Autodesk Inventor part; units mm, degrees
(part 2 of 3)
  line L904 (22.3445, 15.4233) -> (22.5183, 15.4736)
  line L905 (22.5183, 15.4736) -> (22.7031, 15.5229)
  line L906 (22.7031, 15.5229) -> (22.8994, 15.5709)
  line L907 (22.8994, 15.5709) -> (23.1087, 15.6175)
  line L908 (23.1087, 15.6175) -> (23.3298, 15.6619)
  line L909 (23.3298, 15.6619) -> (23.5638, 15.7037)
  line L910 (23.5638, 15.7037) -> (23.7624, 15.7353)
  arc A23 (24.1846, 15.0784) -> (23.7624, 15.7353) centre (0, 0) ccw
  line L911 (24.1846, 15.0784) -> (24.0734, 14.9109)
  line L912 (24.0734, 14.9109) -> (23.9381, 14.7154)
  line L913 (23.9381, 14.7154) -> (23.8059, 14.5327)
  line L914 (23.8059, 14.5327) -> (23.6766, 14.3617)
  line L915 (23.6766, 14.3617) -> (23.5513, 14.203)
  line L916 (23.5513, 14.203) -> (23.4297, 14.0554)
  line L917 (23.4297, 14.0554) -> (23.3117, 13.9182)
  line L918 (23.3117, 13.9182) -> (23.1991, 13.7927)
  line L919 (23.1991, 13.7927) -> (23.0918, 13.6779)
  line L920 (23.0918, 13.6779) -> (22.8926, 13.4778)
  line L921 (22.8926, 13.4778) -> (22.6638, 13.2667)
  line L922 (22.6638, 13.2667) -> (22.6103, 13.2101)
  line L923 (22.6103, 13.2101) -> (22.5689, 13.1572)
  line L924 (22.5689, 13.1572) -> (22.5396, 13.1087)
  line L925 (22.5396, 13.1087) -> (22.5221, 13.0649)
  line L926 (22.5221, 13.0649) -> (22.5162, 13.0264)
  line L927 (22.5162, 13.0264) -> (22.5217, 12.9935)
  line L928 (22.5217, 12.9935) -> (22.5383, 12.9627)
  line L929 (22.5383, 12.9627) -> (22.6394, 12.7851)
  line L930 (22.6394, 12.7851) -> (22.7393, 12.6067)
  line L931 (22.7393, 12.6067) -> (22.7571, 12.5766)
  line L932 (22.7571, 12.5766) -> (22.7824, 12.5549)
  line L933 (22.7824, 12.5549) -> (22.8185, 12.5401)
  line L934 (22.8185, 12.5401) -> (22.865, 12.5325)
  line L935 (22.865, 12.5325) -> (22.9217, 12.5325)
  line L936 (22.9217, 12.5325) -> (22.9883, 12.5406)
  line L937 (22.9883, 12.5406) -> (23.0645, 12.5572)
  line L938 (23.0645, 12.5572) -> (23.3634, 12.6442)
  line L939 (23.3634, 12.6442) -> (23.6375, 12.7114)
  line L940 (23.6375, 12.7114) -> (23.7913, 12.7441)
  line L941 (23.7913, 12.7441) -> (23.9569, 12.7757)
  line L942 (23.9569, 12.7757) -> (24.1353, 12.8058)
  line L943 (24.1353, 12.8058) -> (24.3246, 12.8337)
  line L944 (24.3246, 12.8337) -> (24.5251, 12.8591)
  line L945 (24.5251, 12.8591) -> (24.7384, 12.8815)
  line L946 (24.7384, 12.8815) -> (24.9631, 12.9004)
  line L947 (24.9631, 12.9004) -> (25.2003, 12.9153)
  line L948 (25.2003, 12.9153) -> (25.4012, 12.924)
  arc A24 (25.7457, 12.2232) -> (25.4012, 12.924) centre (0, 0) ccw
  line L949 (25.7457, 12.2232) -> (25.6162, 12.0695)
  line L950 (25.6162, 12.0695) -> (25.4595, 11.8907)
  line L951 (25.4595, 11.8907) -> (25.3073, 11.7243)
  line L952 (25.3073, 11.7243) -> (25.1594, 11.5691)
  line L953 (25.1594, 11.5691) -> (25.0168, 11.4258)
  line L954 (25.0168, 11.4258) -> (24.8791, 11.293)
  line L955 (24.8791, 11.293) -> (24.7463, 11.1701)
  line L956 (24.7463, 11.1701) -> (24.6202, 11.0583)
  line L957 (24.6202, 11.0583) -> (24.5004, 10.9564)
  line L958 (24.5004, 10.9564) -> (24.2797, 10.7804)
  line L959 (24.2797, 10.7804) -> (24.0284, 10.5968)
  line L960 (24.0284, 10.5968) -> (23.9687, 10.5466)
  line L961 (23.9687, 10.5466) -> (23.9216, 10.4988)
  line L962 (23.9216, 10.4988) -> (23.8869, 10.4539)
  line L963 (23.8869, 10.4539) -> (23.8646, 10.4124)
  line L964 (23.8646, 10.4124) -> (23.8543, 10.3748)
  line L965 (23.8543, 10.3748) -> (23.856, 10.3416)
  line L966 (23.856, 10.3416) -> (23.869, 10.309)
  line L967 (23.869, 10.309) -> (23.9492, 10.121)
  line L968 (23.9492, 10.121) -> (24.0281, 9.9324)
  line L969 (24.0281, 9.9324) -> (24.0424, 9.9005)
  line L970 (24.0424, 9.9005) -> (24.0651, 9.8761)
  line L971 (24.0651, 9.8761) -> (24.0992, 9.8572)
  line L972 (24.0992, 9.8572) -> (24.1445, 9.8444)
  line L973 (24.1445, 9.8444) -> (24.2009, 9.8379)
  line L974 (24.2009, 9.8379) -> (24.268, 9.8384)
  line L975 (24.268, 9.8384) -> (24.3456, 9.8462)
  line L976 (24.3456, 9.8462) -> (24.6524, 9.8985)
  line L977 (24.6524, 9.8985) -> (24.9324, 9.9341)
  line L978 (24.9324, 9.9341) -> (25.0889, 9.949)
  line L979 (25.0889, 9.949) -> (25.2571, 9.9615)
  line L980 (25.2571, 9.9615) -> (25.4378, 9.9711)
  line L981 (25.4378, 9.9711) -> (25.6289, 9.9773)
  line L982 (25.6289, 9.9773) -> (25.8311, 9.9796)
  line L983 (25.8311, 9.9796) -> (26.0455, 9.9776)
  line L984 (26.0455, 9.9776) -> (26.2709, 9.9707)
  line L985 (26.2709, 9.9707) -> (26.5083, 9.9585)
  line L986 (26.5083, 9.9585) -> (26.7088, 9.9443)
  arc A25 (26.9713, 9.2088) -> (26.7088, 9.9443) centre (0, 0) ccw
  line L987 (26.9713, 9.2088) -> (26.825, 9.0708)
  line L988 (26.825, 9.0708) -> (26.649, 8.9111)
  line L989 (26.649, 8.9111) -> (26.4788, 8.7631)
  line L990 (26.4788, 8.7631) -> (26.3141, 8.6258)
  line L991 (26.3141, 8.6258) -> (26.1562, 8.4996)
  line L992 (26.1562, 8.4996) -> (26.0043, 8.3834)
  line L993 (26.0043, 8.3834) -> (25.8583, 8.2765)
  line L994 (25.8583, 8.2765) -> (25.7202, 8.1797)
  line L995 (25.7202, 8.1797) -> (25.5896, 8.0922)
  line L996 (25.5896, 8.0922) -> (25.3504, 7.9424)
  line L997 (25.3504, 7.9424) -> (25.0797, 7.7887)
  line L998 (25.0797, 7.7887) -> (25.0147, 7.7456)
  line L999 (25.0147, 7.7456) -> (24.9625, 7.7035)
  line L1000 (24.9625, 7.7035) -> (24.9229, 7.6629)
  line L1001 (24.9229, 7.6629) -> (24.8959, 7.6242)
  line L1002 (24.8959, 7.6242) -> (24.8815, 7.588)
  line L1003 (24.8815, 7.588) -> (24.8794, 7.5548)
  line L1004 (24.8794, 7.5548) -> (24.8885, 7.521)
  line L1005 (24.8885, 7.521) -> (24.9468, 7.325)
  line L1006 (24.9468, 7.325) -> (25.0037, 7.1287)
  line L1007 (25.0037, 7.1287) -> (25.0143, 7.0953)
  line L1008 (25.0143, 7.0953) -> (25.034, 7.0685)
  line L1009 (25.034, 7.0685) -> (25.0657, 7.0459)
  line L1010 (25.0657, 7.0459) -> (25.1093, 7.0279)
  line L1011 (25.1093, 7.0279) -> (25.1646, 7.0151)
  line L1012 (25.1646, 7.0151) -> (25.2313, 7.0079)
  line L1013 (25.2313, 7.0079) -> (25.3092, 7.0069)
  line L1014 (25.3092, 7.0069) -> (25.6201, 7.0238)
  line L1015 (25.6201, 7.0238) -> (25.9023, 7.0272)
  line L1016 (25.9023, 7.0272) -> (26.0595, 7.0242)
  line L1017 (26.0595, 7.0242) -> (26.228, 7.0175)
  line L1018 (26.228, 7.0175) -> (26.4086, 7.0064)
  line L1019 (26.4086, 7.0064) -> (26.5992, 6.9908)
  line L1020 (26.5992, 6.9908) -> (26.8003, 6.97)
  line L1021 (26.8003, 6.97) -> (27.0131, 6.9436)
  line L1022 (27.0131, 6.9436) -> (27.2362, 6.9111)
  line L1023 (27.2362, 6.9111) -> (27.4707, 6.8718)
  line L1024 (27.4707, 6.8718) -> (27.6683, 6.8349)
  arc A26 (27.8452, 6.0743) -> (27.6683, 6.8349) centre (0, 0) ccw
  line L1025 (27.8452, 6.0743) -> (27.6842, 5.9539)
  line L1026 (27.6842, 5.9539) -> (27.4911, 5.8152)
  line L1027 (27.4911, 5.8152) -> (27.3052, 5.6876)
  line L1028 (27.3052, 5.6876) -> (27.1259, 5.57)
  line L1029 (27.1259, 5.57) -> (26.9546, 5.4626)
  line L1030 (26.9546, 5.4626) -> (26.7904, 5.3644)
  line L1031 (26.7904, 5.3644) -> (26.6332, 5.2749)
  line L1032 (26.6332, 5.2749) -> (26.485, 5.1945)
  line L1033 (26.485, 5.1945) -> (26.3453, 5.1224)
  line L1034 (26.3453, 5.1224) -> (26.0905, 5.0009)
  line L1035 (26.0905, 5.0009) -> (25.8041, 4.879)
  line L1036 (25.8041, 4.879) -> (25.7346, 4.8437)
  line L1037 (25.7346, 4.8437) -> (25.6779, 4.8078)
  line L1038 (25.6779, 4.8078) -> (25.6339, 4.7719)
  line L1039 (25.6339, 4.7719) -> (25.6028, 4.7366)
  line L1040 (25.6028, 4.7366) -> (25.5842, 4.7023)
  line L1041 (25.5842, 4.7023) -> (25.5784, 4.6695)
  line L1042 (25.5784, 4.6695) -> (25.5836, 4.6349)
  line L1043 (25.5836, 4.6349) -> (25.6192, 4.4336)
  line L1044 (25.6192, 4.4336) -> (25.6534, 4.232)
  line L1045 (25.6534, 4.232) -> (25.66, 4.1976)
  line L1046 (25.66, 4.1976) -> (25.6766, 4.1688)
  line L1047 (25.6766, 4.1688) -> (25.7055, 4.1427)
  line L1048 (25.7055, 4.1427) -> (25.7468, 4.1199)
  line L1049 (25.7468, 4.1199) -> (25.8002, 4.1008)
  line L1050 (25.8002, 4.1008) -> (25.8657, 4.0861)
  line L1051 (25.8657, 4.0861) -> (25.943, 4.0762)
  line L1052 (25.943, 4.0762) -> (26.2537, 4.0576)
  line L1053 (26.2537, 4.0576) -> (26.5345, 4.0288)
  line L1054 (26.5345, 4.0288) -> (26.6903, 4.0079)
  line L1055 (26.6903, 4.0079) -> (26.857, 3.982)
  line L1056 (26.857, 3.982) -> (27.0351, 3.9504)
  line L1057 (27.0351, 3.9504) -> (27.2227, 3.9131)
  line L1058 (27.2227, 3.9131) -> (27.4201, 3.8696)
  line L1059 (27.4201, 3.8696) -> (27.6285, 3.8191)
  line L1060 (27.6285, 3.8191) -> (27.8465, 3.7613)
  line L1061 (27.8465, 3.7613) -> (28.075, 3.6956)
  line L1062 (28.075, 3.6956) -> (28.2671, 3.6364)
  arc A27 (28.3561, 2.8605) -> (28.2671, 3.6364) centre (0, 0) ccw
  line L1063 (28.3561, 2.8605) -> (28.1824, 2.7593)
  line L1064 (28.1824, 2.7593) -> (27.9748, 2.6436)
  line L1065 (27.9748, 2.6436) -> (27.7755, 2.538)
  line L1066 (27.7755, 2.538) -> (27.584, 2.4415)
  line L1067 (27.584, 2.4415) -> (27.4016, 2.3544)
  line L1068 (27.4016, 2.3544) -> (27.2273, 2.2756)
  line L1069 (27.2273, 2.2756) -> (27.0609, 2.2045)
  line L1070 (27.0609, 2.2045) -> (26.9045, 2.1416)
  line L1071 (26.9045, 2.1416) -> (26.7575, 2.0859)
  line L1072 (26.7575, 2.0859) -> (26.4905, 1.9943)
  line L1073 (26.4905, 1.9943) -> (26.192, 1.9058)
  line L1074 (26.192, 1.9058) -> (26.119, 1.8786)
  line L1075 (26.119, 1.8786) -> (26.0586, 1.8494)
  line L1076 (26.0586, 1.8494) -> (26.0108, 1.8188)
  line L1077 (26.0108, 1.8188) -> (25.9758, 1.7872)
  line L1078 (25.9758, 1.7872) -> (25.9535, 1.7552)
  line L1079 (25.9535, 1.7552) -> (25.9439, 1.7234)
  line L1080 (25.9439, 1.7234) -> (25.9452, 1.6884)
  line L1081 (25.9452, 1.6884) -> (25.9576, 1.4843)
  line L1082 (25.9576, 1.4843) -> (25.9685, 1.2802)
  line L1083 (25.9685, 1.2802) -> (25.9713, 1.2453)
  line L1084 (25.9713, 1.2453) -> (25.9844, 1.2147)
  line L1085 (25.9844, 1.2147) -> (26.0102, 1.1855)
  line L1086 (26.0102, 1.1855) -> (26.0486, 1.1581)
  line L1087 (26.0486, 1.1581) -> (26.0995, 1.1331)
  line L1088 (26.0995, 1.1331) -> (26.1629, 1.111)
  line L1089 (26.1629, 1.111) -> (26.2385, 1.0923)
  line L1090 (26.2385, 1.0923) -> (26.5451, 1.0384)
  line L1091 (26.5451, 1.0384) -> (26.8208, 0.9778)
  line L1092 (26.8208, 0.9778) -> (26.9732, 0.9393)
  line L1093 (26.9732, 0.9393) -> (27.1358, 0.8945)
  line L1094 (27.1358, 0.8945) -> (27.3092, 0.8429)
  line L1095 (27.3092, 0.8429) -> (27.4913, 0.7845)
  line L1096 (27.4913, 0.7845) -> (27.6825, 0.7187)
  line L1097 (27.6825, 0.7187) -> (27.8838, 0.6447)
  line L1098 (27.8838, 0.6447) -> (28.0938, 0.5625)
  line L1099 (28.0938, 0.5625) -> (28.3132, 0.4712)
  line L1100 (28.3132, 0.4712) -> (28.4973, 0.3904)
  arc A28 (28.4973, -0.3904) -> (28.4973, 0.3904) centre (0, 0) ccw
  line L1101 (28.4973, -0.3904) -> (28.3132, -0.4712)
  line L1102 (28.3132, -0.4712) -> (28.0938, -0.5625)
  line L1103 (28.0938, -0.5625) -> (27.8838, -0.6447)
  line L1104 (27.8838, -0.6447) -> (27.6825, -0.7187)
  line L1105 (27.6825, -0.7187) -> (27.4913, -0.7845)
  line L1106 (27.4913, -0.7845) -> (27.3092, -0.8429)
  line L1107 (27.3092, -0.8429) -> (27.1358, -0.8945)
  line L1108 (27.1358, -0.8945) -> (26.9732, -0.9393)
  line L1109 (26.9732, -0.9393) -> (26.8208, -0.9778)
  line L1110 (26.8208, -0.9778) -> (26.5451, -1.0384)
  line L1111 (26.5451, -1.0384) -> (26.2385, -1.0923)
  line L1112 (26.2385, -1.0923) -> (26.1629, -1.111)
  line L1113 (26.1629, -1.111) -> (26.0995, -1.1331)
  line L1114 (26.0995, -1.1331) -> (26.0486, -1.1581)
  line L1115 (26.0486, -1.1581) -> (26.0102, -1.1855)
  line L1116 (26.0102, -1.1855) -> (25.9844, -1.2147)
  line L1117 (25.9844, -1.2147) -> (25.9713, -1.2453)
  line L1118 (25.9713, -1.2453) -> (25.9685, -1.2802)
  line L1119 (25.9685, -1.2802) -> (25.9576, -1.4843)
  line L1120 (25.9576, -1.4843) -> (25.9452, -1.6884)
  line L1121 (25.9452, -1.6884) -> (25.9439, -1.7234)
  line L1122 (25.9439, -1.7234) -> (25.9535, -1.7552)
  line L1123 (25.9535, -1.7552) -> (25.9758, -1.7872)
  line L1124 (25.9758, -1.7872) -> (26.0108, -1.8188)
  line L1125 (26.0108, -1.8188) -> (26.0586, -1.8494)
  line L1126 (26.0586, -1.8494) -> (26.119, -1.8786)
  line L1127 (26.119, -1.8786) -> (26.192, -1.9058)
  line L1128 (26.192, -1.9058) -> (26.4905, -1.9943)
  line L1129 (26.4905, -1.9943) -> (26.7575, -2.0859)
  line L1130 (26.7575, -2.0859) -> (26.9045, -2.1416)
  line L1131 (26.9045, -2.1416) -> (27.0609, -2.2045)
  line L1132 (27.0609, -2.2045) -> (27.2273, -2.2756)
  line L1133 (27.2273, -2.2756) -> (27.4016, -2.3544)
  line L1134 (27.4016, -2.3544) -> (27.584, -2.4415)
  line L1135 (27.584, -2.4415) -> (27.7755, -2.538)
  line L1136 (27.7755, -2.538) -> (27.9748, -2.6436)
  line L1137 (27.9748, -2.6436) -> (28.1824, -2.7593)
  line L1138 (28.1824, -2.7593) -> (28.3561, -2.8605)
  arc A29 (28.2671, -3.6364) -> (28.3561, -2.8605) centre (0, 0) ccw
  line L1139 (28.2671, -3.6364) -> (28.075, -3.6956)
  line L1140 (28.075, -3.6956) -> (27.8465, -3.7613)
  line L1141 (27.8465, -3.7613) -> (27.6285, -3.8191)
  line L1142 (27.6285, -3.8191) -> (27.4201, -3.8696)
  line L1143 (27.4201, -3.8696) -> (27.2227, -3.9131)
  line L1144 (27.2227, -3.9131) -> (27.0351, -3.9504)
  line L1145 (27.0351, -3.9504) -> (26.857, -3.982)
  line L1146 (26.857, -3.982) -> (26.6903, -4.0079)
  line L1147 (26.6903, -4.0079) -> (26.5345, -4.0288)
  line L1148 (26.5345, -4.0288) -> (26.2537, -4.0576)
  line L1149 (26.2537, -4.0576) -> (25.943, -4.0762)
  line L1150 (25.943, -4.0762) -> (25.8657, -4.0861)
  line L1151 (25.8657, -4.0861) -> (25.8002, -4.1008)
  line L1152 (25.8002, -4.1008) -> (25.7468, -4.1199)
  line L1153 (25.7468, -4.1199) -> (25.7055, -4.1427)
  line L1154 (25.7055, -4.1427) -> (25.6766, -4.1688)
  line L1155 (25.6766, -4.1688) -> (25.66, -4.1976)
  line L1156 (25.66, -4.1976) -> (25.6534, -4.232)
  line L1157 (25.6534, -4.232) -> (25.6192, -4.4336)
  line L1158 (25.6192, -4.4336) -> (25.5836, -4.6349)
  line L1159 (25.5836, -4.6349) -> (25.5784, -4.6695)
  line L1160 (25.5784, -4.6695) -> (25.5842, -4.7023)
  line L1161 (25.5842, -4.7023) -> (25.6028, -4.7366)
  line L1162 (25.6028, -4.7366) -> (25.6339, -4.7719)
  line L1163 (25.6339, -4.7719) -> (25.6779, -4.8078)
  line L1164 (25.6779, -4.8078) -> (25.7346, -4.8437)
  line L1165 (25.7346, -4.8437) -> (25.8041, -4.879)
  line L1166 (25.8041, -4.879) -> (26.0905, -5.0009)
  line L1167 (26.0905, -5.0009) -> (26.3453, -5.1224)
  line L1168 (26.3453, -5.1224) -> (26.485, -5.1945)
  line L1169 (26.485, -5.1945) -> (26.6332, -5.2749)
  line L1170 (26.6332, -5.2749) -> (26.7904, -5.3644)
  line L1171 (26.7904, -5.3644) -> (26.9546, -5.4626)
  line L1172 (26.9546, -5.4626) -> (27.1259, -5.57)
  line L1173 (27.1259, -5.57) -> (27.3052, -5.6876)
  line L1174 (27.3052, -5.6876) -> (27.4911, -5.8152)
  line L1175 (27.4911, -5.8152) -> (27.6842, -5.9539)
  line L1176 (27.6842, -5.9539) -> (27.8452, -6.0742)
  arc A30 (27.6683, -6.8349) -> (27.8452, -6.0742) centre (0, 0) ccw
  line L1177 (27.6683, -6.8349) -> (27.4707, -6.8718)
  line L1178 (27.4707, -6.8718) -> (27.2362, -6.9111)
  line L1179 (27.2362, -6.9111) -> (27.0131, -6.9436)
  line L1180 (27.0131, -6.9436) -> (26.8003, -6.97)
  line L1181 (26.8003, -6.97) -> (26.5992, -6.9908)
  line L1182 (26.5992, -6.9908) -> (26.4086, -7.0064)
  line L1183 (26.4086, -7.0064) -> (26.228, -7.0175)
  line L1184 (26.228, -7.0175) -> (26.0595, -7.0242)
  line L1185 (26.0595, -7.0242) -> (25.9023, -7.0272)
  line L1186 (25.9023, -7.0272) -> (25.6201, -7.0238)
  line L1187 (25.6201, -7.0238) -> (25.3092, -7.0069)
  line L1188 (25.3092, -7.0069) -> (25.2313, -7.0079)
  line L1189 (25.2313, -7.0079) -> (25.1646, -7.0151)
  line L1190 (25.1646, -7.0151) -> (25.1093, -7.0279)
  line L1191 (25.1093, -7.0279) -> (25.0657, -7.0459)
  line L1192 (25.0657, -7.0459) -> (25.034, -7.0685)
  line L1193 (25.034, -7.0685) -> (25.0143, -7.0953)
  line L1194 (25.0143, -7.0953) -> (25.0037, -7.1287)
  line L1195 (25.0037, -7.1287) -> (24.9468, -7.325)
  line L1196 (24.9468, -7.325) -> (24.8885, -7.521)
  line L1197 (24.8885, -7.521) -> (24.8794, -7.5548)
  line L1198 (24.8794, -7.5548) -> (24.8815, -7.588)
  line L1199 (24.8815, -7.588) -> (24.8959, -7.6242)
  line L1200 (24.8959, -7.6242) -> (24.9229, -7.6629)
  line L1201 (24.9229, -7.6629) -> (24.9625, -7.7035)
  line L1202 (24.9625, -7.7035) -> (25.0147, -7.7456)
  line L1203 (25.0147, -7.7456) -> (25.0797, -7.7887)
  line L1204 (25.0797, -7.7887) -> (25.3504, -7.9424)
  line L1205 (25.3504, -7.9424) -> (25.5896, -8.0922)
  line L1206 (25.5896, -8.0922) -> (25.7202, -8.1797)
  line L1207 (25.7202, -8.1797) -> (25.8583, -8.2765)
  line L1208 (25.8583, -8.2765) -> (26.0043, -8.3834)
  line L1209 (26.0043, -8.3834) -> (26.1562, -8.4996)
  line L1210 (26.1562, -8.4996) -> (26.3141, -8.6258)
  line L1211 (26.3141, -8.6258) -> (26.4788, -8.7631)
  line L1212 (26.4788, -8.7631) -> (26.649, -8.9111)
  line L1213 (26.649, -8.9111) -> (26.825, -9.0708)
  line L1214 (26.825, -9.0708) -> (26.9713, -9.2088)
  arc A31 (26.7088, -9.9443) -> (26.9713, -9.2088) centre (0, 0) ccw
  line L1215 (26.7088, -9.9443) -> (26.5083, -9.9585)
  line L1216 (26.5083, -9.9585) -> (26.2709, -9.9707)
  line L1217 (26.2709, -9.9707) -> (26.0455, -9.9776)
  line L1218 (26.0455, -9.9776) -> (25.8311, -9.9796)
  line L1219 (25.8311, -9.9796) -> (25.6289, -9.9773)
  line L1220 (25.6289, -9.9773) -> (25.4378, -9.9711)
  line L1221 (25.4378, -9.9711) -> (25.2571, -9.9615)
  line L1222 (25.2571, -9.9615) -> (25.0889, -9.949)
  line L1223 (25.0889, -9.949) -> (24.9324, -9.9341)
  line L1224 (24.9324, -9.9341) -> (24.6524, -9.8985)
  line L1225 (24.6524, -9.8985) -> (24.3456, -9.8462)
  line L1226 (24.3456, -9.8462) -> (24.268, -9.8384)
  line L1227 (24.268, -9.8384) -> (24.2009, -9.8379)
  line L1228 (24.2009, -9.8379) -> (24.1445, -9.8444)
  line L1229 (24.1445, -9.8444) -> (24.0992, -9.8572)
  line L1230 (24.0992, -9.8572) -> (24.0651, -9.8761)
  line L1231 (24.0651, -9.8761) -> (24.0424, -9.9005)
  line L1232 (24.0424, -9.9005) -> (24.0281, -9.9324)
  line L1233 (24.0281, -9.9324) -> (23.9492, -10.121)
  line L1234 (23.9492, -10.121) -> (23.869, -10.309)
  line L1235 (23.869, -10.309) -> (23.856, -10.3416)
  line L1236 (23.856, -10.3416) -> (23.8543, -10.3748)
  line L1237 (23.8543, -10.3748) -> (23.8646, -10.4124)
  line L1238 (23.8646, -10.4124) -> (23.8869, -10.4539)
  line L1239 (23.8869, -10.4539) -> (23.9216, -10.4988)
  line L1240 (23.9216, -10.4988) -> (23.9687, -10.5466)
  line L1241 (23.9687, -10.5466) -> (24.0284, -10.5968)
  line L1242 (24.0284, -10.5968) -> (24.2797, -10.7804)
  line L1243 (24.2797, -10.7804) -> (24.5004, -10.9564)
  line L1244 (24.5004, -10.9564) -> (24.6202, -11.0583)
  line L1245 (24.6202, -11.0583) -> (24.7463, -11.1701)
  line L1246 (24.7463, -11.1701) -> (24.8791, -11.293)
  line L1247 (24.8791, -11.293) -> (25.0168, -11.4258)
  line L1248 (25.0168, -11.4258) -> (25.1594, -11.5691)
  line L1249 (25.1594, -11.5691) -> (25.3073, -11.7243)
  line L1250 (25.3073, -11.7243) -> (25.4595, -11.8907)
  line L1251 (25.4595, -11.8907) -> (25.6162, -12.0695)
  line L1252 (25.6162, -12.0695) -> (25.7457, -12.2232)
  arc A32 (25.4012, -12.924) -> (25.7457, -12.2232) centre (0, 0) ccw
  line L1253 (25.4012, -12.924) -> (25.2003, -12.9153)
  line L1254 (25.2003, -12.9153) -> (24.9631, -12.9004)
  line L1255 (24.9631, -12.9004) -> (24.7384, -12.8815)
  line L1256 (24.7384, -12.8815) -> (24.5251, -12.8591)
  line L1257 (24.5251, -12.8591) -> (24.3246, -12.8337)
  line L1258 (24.3246, -12.8337) -> (24.1353, -12.8058)
  line L1259 (24.1353, -12.8058) -> (23.9569, -12.7757)
  line L1260 (23.9569, -12.7757) -> (23.7913, -12.7441)
  line L1261 (23.7913, -12.7441) -> (23.6375, -12.7114)
  line L1262 (23.6375, -12.7114) -> (23.3634, -12.6442)
  line L1263 (23.3634, -12.6442) -> (23.0645, -12.5572)
  line L1264 (23.0645, -12.5572) -> (22.9883, -12.5406)
  line L1265 (22.9883, -12.5406) -> (22.9217, -12.5325)
  line L1266 (22.9217, -12.5325) -> (22.865, -12.5325)
  line L1267 (22.865, -12.5325) -> (22.8185, -12.5401)
  line L1268 (22.8185, -12.5401) -> (22.7824, -12.5549)
  line L1269 (22.7824, -12.5549) -> (22.7571, -12.5766)
  line L1270 (22.7571, -12.5766) -> (22.7393, -12.6067)
  line L1271 (22.7393, -12.6067) -> (22.6394, -12.7851)
  line L1272 (22.6394, -12.7851) -> (22.5383, -12.9627)
  line L1273 (22.5383, -12.9627) -> (22.5217, -12.9935)
  line L1274 (22.5217, -12.9935) -> (22.5162, -13.0264)
  line L1275 (22.5162, -13.0264) -> (22.5221, -13.0649)
  line L1276 (22.5221, -13.0649) -> (22.5396, -13.1087)
  line L1277 (22.5396, -13.1087) -> (22.5689, -13.1572)
  line L1278 (22.5689, -13.1572) -> (22.6103, -13.2101)
  line L1279 (22.6103, -13.2101) -> (22.6638, -13.2667)
  line L1280 (22.6638, -13.2667) -> (22.8926, -13.4778)
  line L1281 (22.8926, -13.4778) -> (23.0918, -13.6779)
  line L1282 (23.0918, -13.6779) -> (23.1991, -13.7927)
  line L1283 (23.1991, -13.7927) -> (23.3117, -13.9182)
  line L1284 (23.3117, -13.9182) -> (23.4297, -14.0554)
  line L1285 (23.4297, -14.0554) -> (23.5513, -14.203)
  line L1286 (23.5513, -14.203) -> (23.6766, -14.3617)
  line L1287 (23.6766, -14.3617) -> (23.8059, -14.5327)
  line L1288 (23.8059, -14.5327) -> (23.9381, -14.7154)
  line L1289 (23.9381, -14.7154) -> (24.0734, -14.9109)
  line L1290 (24.0734, -14.9109) -> (24.1846, -15.0784)
  arc A33 (23.7624, -15.7353) -> (24.1846, -15.0784) centre (0, 0) ccw
  line L1291 (23.7624, -15.7353) -> (23.5638, -15.7037)
  line L1292 (23.5638, -15.7037) -> (23.3298, -15.6619)
  line L1293 (23.3298, -15.6619) -> (23.1087, -15.6175)
  line L1294 (23.1087, -15.6175) -> (22.8994, -15.5709)
  line L1295 (22.8994, -15.5709) -> (22.7031, -15.5229)
  line L1296 (22.7031, -15.5229) -> (22.5183, -15.4736)
  line L1297 (22.5183, -15.4736) -> (22.3445, -15.4233)
  line L1298 (22.3445, -15.4233) -> (22.1835, -15.373)
  line L1299 (22.1835, -15.373) -> (22.0345, -15.323)
  line L1300 (22.0345, -15.323) -> (21.7698, -15.225)
  line L1301 (21.7698, -15.225) -> (21.4827, -15.1045)
  line L1302 (21.4827, -15.1045) -> (21.4089, -15.0794)
  line L1303 (21.4089, -15.0794) -> (21.3437, -15.0637)
  line L1304 (21.3437, -15.0637) -> (21.2874, -15.0572)
  line L1305 (21.2874, -15.0572) -> (21.2403, -15.0594)
  line L1306 (21.2403, -15.0594) -> (21.2028, -15.0701)
  line L1307 (21.2028, -15.0701) -> (21.1752, -15.0887)
  line L1308 (21.1752, -15.0887) -> (21.154, -15.1166)
  line L1309 (21.154, -15.1166) -> (21.0344, -15.2824)
  line L1310 (21.0344, -15.2824) -> (20.9137, -15.4474)
  line L1311 (20.9137, -15.4474) -> (20.8937, -15.4761)
  line L1312 (20.8937, -15.4761) -> (20.8845, -15.5081)
  line L1313 (20.8845, -15.5081) -> (20.886, -15.5471)
  line L1314 (20.886, -15.5471) -> (20.8984, -15.5926)
  line L1315 (20.8984, -15.5926) -> (20.922, -15.6441)
  line L1316 (20.922, -15.6441) -> (20.957, -15.7013)
  line L1317 (20.957, -15.7013) -> (21.0038, -15.7637)
  line L1318 (21.0038, -15.7637) -> (21.207, -15.9995)
  line L1319 (21.207, -15.9995) -> (21.3821, -16.221)
  line L1320 (21.3821, -16.221) -> (21.4757, -16.3473)
  line L1321 (21.4757, -16.3473) -> (21.5732, -16.4848)
  line L1322 (21.5732, -16.4848) -> (21.6748, -16.6345)
  line L1323 (21.6748, -16.6345) -> (21.7788, -16.7951)
  line L1324 (21.7788, -16.7951) -> (21.8851, -16.967)
  line L1325 (21.8851, -16.967) -> (21.9941, -17.1517)
  line L1326 (21.9941, -17.1517) -> (22.1046, -17.3482)
  line L1327 (22.1046, -17.3482) -> (22.2167, -17.5578)
  line L1328 (22.2167, -17.5578) -> (22.3081, -17.7369)
  arc A34 (21.8138, -18.3414) -> (22.3081, -17.7369) centre (0, 0) ccw
  line L1329 (21.8138, -18.3414) -> (21.6202, -18.2874)
  line L1330 (21.6202, -18.2874) -> (21.3925, -18.2192)
  line L1331 (21.3925, -18.2192) -> (21.1779, -18.1499)
  line L1332 (21.1779, -18.1499) -> (20.9752, -18.0798)
  line L1333 (20.9752, -18.0798) -> (20.7856, -18.0097)
  line L1334 (20.7856, -18.0097) -> (20.6076, -17.9396)
  line L1335 (20.6076, -17.9396) -> (20.4407, -17.8698)
  line L1336 (20.4407, -17.8698) -> (20.2865, -17.8015)
  line L1337 (20.2865, -17.8015) -> (20.1442, -17.7349)
  line L1338 (20.1442, -17.7349) -> (19.8924, -17.6073)
  line L1339 (19.8924, -17.6073) -> (19.6209, -17.4549)
  line L1340 (19.6209, -17.4549) -> (19.5505, -17.4215)
  line L1341 (19.5505, -17.4215) -> (19.4874, -17.3985)
  line L1342 (19.4874, -17.3985) -> (19.4322, -17.3856)
  line L1343 (19.4322, -17.3856) -> (19.3852, -17.3825)
  line L1344 (19.3852, -17.3825) -> (19.3467, -17.3888)
  line L1345 (19.3467, -17.3888) -> (19.3172, -17.4041)
  line L1346 (19.3172, -17.4041) -> (19.293, -17.4295)
  line L1347 (19.293, -17.4295) -> (19.1553, -17.5805)
  line L1348 (19.1553, -17.5805) -> (19.0165, -17.7307)
  line L1349 (19.0165, -17.7307) -> (18.9934, -17.757)
  line L1350 (18.9934, -17.757) -> (18.9806, -17.7877)
  line L1351 (18.9806, -17.7877) -> (18.9776, -17.8266)
  line L1352 (18.9776, -17.8266) -> (18.9847, -17.8732)
  line L1353 (18.9847, -17.8732) -> (19.0023, -17.9271)
  line L1354 (19.0023, -17.9271) -> (19.0306, -17.9879)
  line L1355 (19.0306, -17.9879) -> (19.07, -18.0552)
  line L1356 (19.07, -18.0552) -> (19.245, -18.3126)
  line L1357 (19.245, -18.3126) -> (19.3937, -18.5526)
  line L1358 (19.3937, -18.5526) -> (19.4722, -18.6887)
  line L1359 (19.4722, -18.6887) -> (19.5535, -18.8365)
  line L1360 (19.5535, -18.8365) -> (19.6373, -18.9968)
  line L1361 (19.6373, -18.9968) -> (19.7223, -19.1682)
  line L1362 (19.7223, -19.1682) -> (19.8084, -19.3511)
  line L1363 (19.8084, -19.3511) -> (19.8956, -19.547)
  line L1364 (19.8956, -19.547) -> (19.983, -19.7549)
  line L1365 (19.983, -19.7549) -> (20.0705, -19.9759)
  line L1366 (20.0705, -19.9759) -> (20.1409, -20.1642)
  arc A35 (19.5809, -20.7085) -> (20.1409, -20.1642) centre (0, 0) ccw
  line L1367 (19.5809, -20.7085) -> (19.3946, -20.6327)
  line L1368 (19.3946, -20.6327) -> (19.1762, -20.539)
  line L1369 (19.1762, -20.539) -> (18.9709, -20.4457)
  line L1370 (18.9709, -20.4457) -> (18.7776, -20.3529)
  line L1371 (18.7776, -20.3529) -> (18.5972, -20.2616)
  line L1372 (18.5972, -20.2616) -> (18.4283, -20.1717)
  line L1373 (18.4283, -20.1717) -> (18.2705, -20.0834)
  line L1374 (18.2705, -20.0834) -> (18.1251, -19.998)
  line L1375 (18.1251, -19.998) -> (17.9912, -19.9155)
  line L1376 (17.9912, -19.9155) -> (17.7556, -19.7601)
  line L1377 (17.7556, -19.7601) -> (17.5033, -19.5778)
  line L1378 (17.5033, -19.5778) -> (17.4371, -19.5365)
  line L1379 (17.4371, -19.5365) -> (17.3771, -19.5065)
  line L1380 (17.3771, -19.5065) -> (17.3237, -19.4874)
  line L1381 (17.3237, -19.4874) -> (17.2774, -19.4789)
  line L1382 (17.2774, -19.4789) -> (17.2384, -19.4808)
  line L1383 (17.2384, -19.4808) -> (17.2073, -19.4927)
  line L1384 (17.2073, -19.4927) -> (17.1804, -19.5151)
  line L1385 (17.1804, -19.5151) -> (17.0264, -19.6495)
  line L1386 (17.0264, -19.6495) -> (16.8714, -19.7828)
  line L1387 (16.8714, -19.7828) -> (16.8454, -19.8063)
  line L1388 (16.8454, -19.8063) -> (16.8292, -19.8354)
  line L1389 (16.8292, -19.8354) -> (16.8218, -19.8736)
  line L1390 (16.8218, -19.8736) -> (16.8236, -19.9208)
  line L1391 (16.8236, -19.9208) -> (16.8349, -19.9763)
  line L1392 (16.8349, -19.9763) -> (16.8561, -20.04)
  line L1393 (16.8561, -20.04) -> (16.8875, -20.1113)
  line L1394 (16.8875, -20.1113) -> (17.0321, -20.387)
  line L1395 (17.0321, -20.387) -> (17.1524, -20.6424)
  line L1396 (17.1524, -20.6424) -> (17.215, -20.7866)
  line L1397 (17.215, -20.7866) -> (17.2788, -20.9427)
  line L1398 (17.2788, -20.9427) -> (17.3438, -21.1115)
  line L1399 (17.3438, -21.1115) -> (17.4088, -21.2914)
  line L1400 (17.4088, -21.2914) -> (17.4734, -21.483)
  line L1401 (17.4734, -21.483) -> (17.5377, -21.6875)
  line L1402 (17.5377, -21.6875) -> (17.6009, -21.904)
  line L1403 (17.6009, -21.904) -> (17.6626, -22.1336)
  line L1404 (17.6626, -22.1336) -> (17.711, -22.3287)
  arc A36 (17.0926, -22.8055) -> (17.711, -22.3287) centre (0, 0) ccw
  line L1405 (17.0926, -22.8055) -> (16.9163, -22.7091)
  line L1406 (16.9163, -22.7091) -> (16.7099, -22.591)
  line L1407 (16.7099, -22.591) -> (16.5166, -22.4749)
  line L1408 (16.5166, -22.4749) -> (16.3351, -22.3607)
  line L1409 (16.3351, -22.3607) -> (16.1663, -22.2495)
  line L1410 (16.1663, -22.2495) -> (16.0088, -22.1409)
  line L1411 (16.0088, -22.1409) -> (15.862, -22.0352)
  line L1412 (15.862, -22.0352) -> (15.7273, -21.9337)
  line L1413 (15.7273, -21.9337) -> (15.6038, -21.8366)
  line L1414 (15.6038, -21.8366) -> (15.3874, -21.6553)
  line L1415 (15.3874, -21.6553) -> (15.1575, -21.4454)
  line L1416 (15.1575, -21.4454) -> (15.0965, -21.3969)
  line L1417 (15.0965, -21.3969) -> (15.0403, -21.3602)
  line L1418 (15.0403, -21.3602) -> (14.9894, -21.3351)
  line L1419 (14.9894, -21.3351) -> (14.9443, -21.3214)
  line L1420 (14.9443, -21.3214) -> (14.9054, -21.3189)
  line L1421 (14.9054, -21.3189) -> (14.8732, -21.3271)
  line L1422 (14.8732, -21.3271) -> (14.8439, -21.3463)
  line L1423 (14.8439, -21.3463) -> (14.6755, -21.4623)
  line L1424 (14.6755, -21.4623) -> (14.5064, -21.5771)
  line L1425 (14.5064, -21.5771) -> (14.4779, -21.5974)
  line L1426 (14.4779, -21.5974) -> (14.4585, -21.6245)
  line L1427 (14.4585, -21.6245) -> (14.4468, -21.6616)
  line L1428 (14.4468, -21.6616) -> (14.4432, -21.7086)
  line L1429 (14.4432, -21.7086) -> (14.4481, -21.7652)
  line L1430 (14.4481, -21.7652) -> (14.4618, -21.8308)
  line L1431 (14.4618, -21.8308) -> (14.4849, -21.9053)
  line L1432 (14.4849, -21.9053) -> (14.5971, -22.1957)
  line L1433 (14.5971, -22.1957) -> (14.6875, -22.463)
  line L1434 (14.6875, -22.463) -> (14.7333, -22.6135)
  line L1435 (14.7333, -22.6135) -> (14.7789, -22.7758)
  line L1436 (14.7789, -22.7758) -> (14.8242, -22.9509)
  line L1437 (14.8242, -22.9509) -> (14.8682, -23.1371)
  line L1438 (14.8682, -23.1371) -> (14.9106, -23.3347)
  line L1439 (14.9106, -23.3347) -> (14.9512, -23.5453)
  line L1440 (14.9512, -23.5453) -> (14.9893, -23.7676)
  line L1441 (14.9893, -23.7676) -> (15.0244, -24.0027)
  line L1442 (15.0244, -24.0027) -> (15.0503, -24.202)
  arc A37 (14.3816, -24.6053) -> (15.0503, -24.202) centre (0, 0) ccw
  line L1443 (14.3816, -24.6053) -> (14.2173, -24.4894)
  line L1444 (14.2173, -24.4894) -> (14.0258, -24.3485)
  line L1445 (14.0258, -24.3485) -> (13.847, -24.2112)
  line L1446 (13.847, -24.2112) -> (13.6797, -24.077)
  line L1447 (13.6797, -24.077) -> (13.5247, -23.9473)
  line L1448 (13.5247, -23.9473) -> (13.3806, -23.8215)
  line L1449 (13.3806, -23.8215) -> (13.2468, -23.6997)
  line L1450 (13.2468, -23.6997) -> (13.1246, -23.5835)
  line L1451 (13.1246, -23.5835) -> (13.0129, -23.4729)
  line L1452 (13.0129, -23.4729) -> (12.8186, -23.2682)
  line L1453 (12.8186, -23.2682) -> (12.6141, -23.0334)
  line L1454 (12.6141, -23.0334) -> (12.559, -22.9783)
  line L1455 (12.559, -22.9783) -> (12.5074, -22.9354)
  line L1456 (12.5074, -22.9354) -> (12.4597, -22.9047)
  line L1457 (12.4597, -22.9047) -> (12.4164, -22.886)
  line L1458 (12.4164, -22.886) -> (12.3781, -22.879)
  line L1459 (12.3781, -22.879) -> (12.3451, -22.8835)
  line L1460 (12.3451, -22.8835) -> (12.3138, -22.8992)
  line L1461 (12.3138, -22.8992) -> (12.1334, -22.9953)
  line L1462 (12.1334, -22.9953) -> (11.9522, -23.09)
  line L1463 (11.9522, -23.09) -> (11.9216, -23.107)
  line L1464 (11.9216, -23.107) -> (11.8992, -23.1316)
  line L1465 (11.8992, -23.1316) -> (11.8834, -23.1673)
  line L1466 (11.8834, -23.1673) -> (11.8744, -23.2135)
  line L1467 (11.8744, -23.2135) -> (11.8728, -23.2702)
  line L1468 (11.8728, -23.2702) -> (11.8791, -23.337)
  line L1469 (11.8791, -23.337) -> (11.8935, -23.4137)
  line L1470 (11.8935, -23.4137) -> (11.9718, -23.7149)
  line L1471 (11.9718, -23.7149) -> (12.0312, -23.9909)
  line L1472 (12.0312, -23.9909) -> (12.0595, -24.1455)
  line L1473 (12.0595, -24.1455) -> (12.0863, -24.312)
  line L1474 (12.0863, -24.312) -> (12.1114, -24.4912)
  line L1475 (12.1114, -24.4912) -> (12.1339, -24.6811)
  line L1476 (12.1339, -24.6811) -> (12.1535, -24.8823)
  line L1477 (12.1535, -24.8823) -> (12.1698, -25.0961)
  line L1478 (12.1698, -25.0961) -> (12.1823, -25.3213)
  line L1479 (12.1823, -25.3213) -> (12.1904, -25.5589)
  line L1480 (12.1904, -25.5589) -> (12.1934, -25.7599)
  arc A38 (11.4831, -26.0843) -> (12.1934, -25.7599) centre (0, 0) ccw
  line L1481 (11.4831, -26.0843) -> (11.3331, -25.9504)
  line L1482 (11.3331, -25.9504) -> (11.1589, -25.7887)
  line L1483 (11.1589, -25.7887) -> (10.9969, -25.6318)
  line L1484 (10.9969, -25.6318) -> (10.846, -25.4795)
  line L1485 (10.846, -25.4795) -> (10.7067, -25.3329)
  line L1486 (10.7067, -25.3329) -> (10.5779, -25.1915)
  line L1487 (10.5779, -25.1915) -> (10.4589, -25.0552)
  line L1488 (10.4589, -25.0552) -> (10.3507, -24.9259)
  line L1489 (10.3507, -24.9259) -> (10.2523, -24.8033)
  line L1490 (10.2523, -24.8033) -> (10.0827, -24.5777)
  line L1491 (10.0827, -24.5777) -> (9.9063, -24.3212)
  line L1492 (9.9063, -24.3212) -> (9.8578, -24.2601)
  line L1493 (9.8578, -24.2601) -> (9.8114, -24.2117)
  line L1494 (9.8114, -24.2117) -> (9.7675, -24.1757)
  line L1495 (9.7675, -24.1757) -> (9.7267, -24.1522)
  line L1496 (9.7267, -24.1522) -> (9.6894, -24.1408)
  line L1497 (9.6894, -24.1408) -> (9.6561, -24.1416)
  line L1498 (9.6561, -24.1416) -> (9.6232, -24.1536)
  line L1499 (9.6232, -24.1536) -> (9.433, -24.2285)
  line L1500 (9.433, -24.2285) -> (9.2422, -24.302)
  line L1501 (9.2422, -24.302) -> (9.2099, -24.3153)
  line L1502 (9.2099, -24.3153) -> (9.1849, -24.3373)
  line L1503 (9.1849, -24.3373) -> (9.165, -24.3708)
  line L1504 (9.165, -24.3708) -> (9.1509, -24.4158)
  line L1505 (9.1509, -24.4158) -> (9.1428, -24.472)
  line L1506 (9.1428, -24.472) -> (9.1414, -24.539)
  line L1507 (9.1414, -24.539) -> (9.147, -24.6168)
  line L1508 (9.147, -24.6168) -> (9.1905, -24.925)
  line L1509 (9.1905, -24.925) -> (9.218, -25.206)
  line L1510 (9.218, -25.206) -> (9.2285, -25.3628)
  line L1511 (9.2285, -25.3628) -> (9.2362, -25.5313)
  line L1512 (9.2362, -25.5313) -> (9.2407, -25.7121)
  line L1513 (9.2407, -25.7121) -> (9.2414, -25.9034)
  line L1514 (9.2414, -25.9034) -> (9.2379, -26.1055)
  line L1515 (9.2379, -26.1055) -> (9.2297, -26.3198)
  line L1516 (9.2297, -26.3198) -> (9.2164, -26.5449)
  line L1517 (9.2164, -26.5449) -> (9.1974, -26.7819)
  line L1518 (9.1974, -26.7819) -> (9.1775, -26.9819)
  arc A39 (8.4348, -27.2232) -> (9.1775, -26.9819) centre (0, 0) ccw
  line L1519 (8.4348, -27.2232) -> (8.3011, -27.0731)
  line L1520 (8.3011, -27.0731) -> (8.1465, -26.8926)
  line L1521 (8.1465, -26.8926) -> (8.0034, -26.7183)
  line L1522 (8.0034, -26.7183) -> (7.8708, -26.5497)
  line L1523 (7.8708, -26.5497) -> (7.7492, -26.3882)
  line L1524 (7.7492, -26.3882) -> (7.6374, -26.2331)
  line L1525 (7.6374, -26.2331) -> (7.5347, -26.0841)
  line L1526 (7.5347, -26.0841) -> (7.4419, -25.9433)
  line L1527 (7.4419, -25.9433) -> (7.3581, -25.8103)
  line L1528 (7.3581, -25.8103) -> (7.2153, -25.5668)
  line L1529 (7.2153, -25.5668) -> (7.0693, -25.2919)
  line L1530 (7.0693, -25.2919) -> (7.0281, -25.2257)
  line L1531 (7.0281, -25.2257) -> (6.9875, -25.1723)
  line L1532 (6.9875, -25.1723) -> (6.948, -25.1316)
  line L1533 (6.948, -25.1316) -> (6.9102, -25.1035)
  line L1534 (6.9102, -25.1035) -> (6.8744, -25.088)
  line L1535 (6.8744, -25.088) -> (6.8413, -25.0849)
  line L1536 (6.8413, -25.0849) -> (6.8072, -25.0932)
  line L1537 (6.8072, -25.0932) -> (6.6097, -25.1458)
  line L1538 (6.6097, -25.1458) -> (6.4118, -25.1971)
  line L1539 (6.4118, -25.1971) -> (6.3781, -25.2067)
  line L1540 (6.3781, -25.2067) -> (6.3507, -25.2256)
  line L1541 (6.3507, -25.2256) -> (6.3272, -25.2567)
  line L1542 (6.3272, -25.2567) -> (6.308, -25.2998)
  line L1543 (6.308, -25.2998) -> (6.2937, -25.3546)
  line L1544 (6.2937, -25.3546) -> (6.2846, -25.4211)
  line L1545 (6.2846, -25.4211) -> (6.2813, -25.499)
  line L1546 (6.2813, -25.499) -> (6.2894, -25.8102)
  line L1547 (6.2894, -25.8102) -> (6.2847, -26.0924)
  line L1548 (6.2847, -26.0924) -> (6.2772, -26.2495)
  line L1549 (6.2772, -26.2495) -> (6.2656, -26.4177)
  line L1550 (6.2656, -26.4177) -> (6.2495, -26.5979)
  line L1551 (6.2495, -26.5979) -> (6.2284, -26.788)
  line L1552 (6.2284, -26.788) -> (6.2019, -26.9884)
  line L1553 (6.2019, -26.9884) -> (6.1694, -27.2004)
  line L1554 (6.1694, -27.2004) -> (6.1305, -27.4225)
  line L1555 (6.1305, -27.4225) -> (6.0846, -27.6557)
  line L1556 (6.0846, -27.6557) -> (6.042, -27.8522)
  arc A40 (5.2766, -28.0073) -> (6.042, -27.8522) centre (0, 0) ccw
  line L1557 (5.2766, -28.0073) -> (5.1609, -27.8429)
  line L1558 (5.1609, -27.8429) -> (5.0278, -27.6459)
  line L1559 (5.0278, -27.6459) -> (4.9055, -27.4564)
  line L1560 (4.9055, -27.4564) -> (4.7931, -27.2739)
  line L1561 (4.7931, -27.2739) -> (4.6907, -27.0996)
  line L1562 (4.6907, -27.0996) -> (4.5972, -26.9327)
  line L1563 (4.5972, -26.9327) -> (4.5122, -26.773)
  line L1564 (4.5122, -26.773) -> (4.4361, -26.6225)
  line L1565 (4.4361, -26.6225) -> (4.368, -26.4808)
  line L1566 (4.368, -26.4808) -> (4.2539, -26.2227)
  line L1567 (4.2539, -26.2227) -> (4.1402, -25.9329)
  line L1568 (4.1402, -25.9329) -> (4.1068, -25.8624)
  line L1569 (4.1068, -25.8624) -> (4.0726, -25.8047)
  line L1570 (4.0726, -25.8047) -> (4.038, -25.7598)
  line L1571 (4.038, -25.7598) -> (4.0035, -25.7276)
  line L1572 (4.0035, -25.7276) -> (3.9698, -25.7081)
  line L1573 (3.9698, -25.7081) -> (3.9372, -25.7013)
  line L1574 (3.9372, -25.7013) -> (3.9024, -25.7056)
  line L1575 (3.9024, -25.7056) -> (3.7002, -25.7354)
  line L1576 (3.7002, -25.7354) -> (3.4977, -25.7637)
  line L1577 (3.4977, -25.7637) -> (3.4632, -25.7694)
  line L1578 (3.4632, -25.7694) -> (3.4338, -25.7851)
  line L1579 (3.4338, -25.7851) -> (3.4069, -25.8133)
  line L1580 (3.4069, -25.8133) -> (3.383, -25.8539)
  line L1581 (3.383, -25.8539) -> (3.3624, -25.9068)
  line L1582 (3.3624, -25.9068) -> (3.3458, -25.9718)
  line L1583 (3.3458, -25.9718) -> (3.3337, -26.0488)
  line L1584 (3.3337, -26.0488) -> (3.3062, -26.3589)
  line L1585 (3.3062, -26.3589) -> (3.2694, -26.6388)
  line L1586 (3.2694, -26.6388) -> (3.2441, -26.7939)
  line L1587 (3.2441, -26.7939) -> (3.2134, -26.9597)
  line L1588 (3.2134, -26.9597) -> (3.1768, -27.1369)
  line L1589 (3.1768, -27.1369) -> (3.1342, -27.3234)
  line L1590 (3.1342, -27.3234) -> (3.085, -27.5195)
  line L1591 (3.085, -27.5195) -> (3.0285, -27.7263)
  line L1592 (3.0285, -27.7263) -> (2.9646, -27.9426)
  line L1593 (2.9646, -27.9426) -> (2.8924, -28.169)
  line L1594 (2.8924, -28.169) -> (2.8277, -28.3594)
  arc A41 (2.0496, -28.4262) -> (2.8277, -28.3594) centre (0, 0) ccw
  line L1595 (2.0496, -28.4262) -> (1.9534, -28.2497)
  line L1596 (1.9534, -28.2497) -> (1.8437, -28.0388)
  line L1597 (1.8437, -28.0388) -> (1.7438, -27.8367)
  line L1598 (1.7438, -27.8367) -> (1.6529, -27.6425)
  line L1599 (1.6529, -27.6425) -> (1.571, -27.4576)
  line L1600 (1.571, -27.4576) -> (1.4972, -27.2812)
  line L1601 (1.4972, -27.2812) -> (1.4309, -27.1128)
  line L1602 (1.4309, -27.1128) -> (1.3724, -26.9547)
  line L1603 (1.3724, -26.9547) -> (1.321, -26.8061)
  line L1604 (1.321, -26.8061) -> (1.237, -26.5366)
  line L1605 (1.237, -26.5366) -> (1.1571, -26.2358)
  line L1606 (1.1571, -26.2358) -> (1.132, -26.162)
  line L1607 (1.132, -26.162) -> (1.1045, -26.1007)
  line L1608 (1.1045, -26.1007) -> (1.0753, -26.0521)
  line L1609 (1.0753, -26.0521) -> (1.0447, -26.0162)
  line L1610 (1.0447, -26.0162) -> (1.0134, -25.993)
  line L1611 (1.0134, -25.993) -> (0.9818, -25.9826)
  line L1612 (0.9818, -25.9826) -> (0.9468, -25.9828)
  line L1613 (0.9468, -25.9828) -> (0.7425, -25.9894)
  line L1614 (0.7425, -25.9894) -> (0.5381, -25.9945)
  line L1615 (0.5381, -25.9945) -> (0.5031, -25.9962)
  line L1616 (0.5031, -25.9962) -> (0.4722, -26.0085)
  line L1617 (0.4722, -26.0085) -> (0.4422, -26.0335)
  line L1618 (0.4422, -26.0335) -> (0.4138, -26.071)
  line L1619 (0.4138, -26.071) -> (0.3873, -26.1212)
  line L1620 (0.3873, -26.1212) -> (0.3634, -26.1839)
  line L1621 (0.3634, -26.1839) -> (0.3426, -26.259)
  line L1622 (0.3426, -26.259) -> (0.28, -26.564)
  line L1623 (0.28, -26.564) -> (0.2115, -26.8378)
  line L1624 (0.2115, -26.8378) -> (0.1686, -26.9891)
  line L1625 (0.1686, -26.9891) -> (0.1193, -27.1503)
  line L1626 (0.1193, -27.1503) -> (0.0627, -27.3221)
  line L1627 (0.0627, -27.3221) -> (-0.0009, -27.5025)
  line L1628 (-0.0009, -27.5025) -> (-0.0721, -27.6917)
  line L1629 (-0.0721, -27.6917) -> (-0.1518, -27.8908)
  line L1630 (-0.1518, -27.8908) -> (-0.2399, -28.0984)
  line L1631 (-0.2399, -28.0984) -> (-0.3375, -28.3151)
  line L1632 (-0.3375, -28.3151) -> (-0.4235, -28.4969)
  arc A42 (-1.2041, -28.4746) -> (-0.4235, -28.4969) centre (0, 0) ccw
  line L1633 (-1.2041, -28.4746) -> (-1.2795, -28.2882)
  line L1634 (-1.2795, -28.2882) -> (-1.3645, -28.0662)
  line L1635 (-1.3645, -28.0662) -> (-1.4407, -27.854)
  line L1636 (-1.4407, -27.854) -> (-1.5089, -27.6507)
  line L1637 (-1.5089, -27.6507) -> (-1.5692, -27.4577)
  line L1638 (-1.5692, -27.4577) -> (-1.6224, -27.274)
  line L1639 (-1.6224, -27.274) -> (-1.6691, -27.0992)
  line L1640 (-1.6691, -27.0992) -> (-1.7091, -26.9354)
  line L1641 (-1.7091, -26.9354) -> (-1.7433, -26.782)
  line L1642 (-1.7433, -26.782) -> (-1.796, -26.5047)
  line L1643 (-1.796, -26.5047) -> (-1.8411, -26.1967)
  line L1644 (-1.8411, -26.1967) -> (-1.8577, -26.1205)
  line L1645 (-1.8577, -26.1205) -> (-1.8779, -26.0565)
  line L1646 (-1.8779, -26.0565) -> (-1.9015, -26.0049)
  line L1647 (-1.9015, -26.0049) -> (-1.9277, -25.9657)
  line L1648 (-1.9277, -25.9657) -> (-1.9562, -25.9391)
  line L1649 (-1.9562, -25.9391) -> (-1.9864, -25.9251)
  line L1650 (-1.9864, -25.9251) -> (-2.0212, -25.9214)
  line L1651 (-2.0212, -25.9214) -> (-2.225, -25.9046)
  line L1652 (-2.225, -25.9046) -> (-2.4286, -25.8864)
  line L1653 (-2.4286, -25.8864) -> (-2.4635, -25.8841)
  line L1654 (-2.4635, -25.8841) -> (-2.4957, -25.8928)
  line L1655 (-2.4957, -25.8928) -> (-2.5282, -25.9142)
  line L1656 (-2.5282, -25.9142) -> (-2.5608, -25.9483)
  line L1657 (-2.5608, -25.9483) -> (-2.5928, -25.9951)
  line L1658 (-2.5928, -25.9951) -> (-2.6237, -26.0547)
  line L1659 (-2.6237, -26.0547) -> (-2.6529, -26.1269)
  line L1660 (-2.6529, -26.1269) -> (-2.7499, -26.4227)
  line L1661 (-2.7499, -26.4227) -> (-2.8492, -26.687)
  line L1662 (-2.8492, -26.687) -> (-2.909, -26.8324)
  line L1663 (-2.909, -26.8324) -> (-2.9764, -26.9869)
  line L1664 (-2.9764, -26.9869) -> (-3.0522, -27.1512)
  line L1665 (-3.0522, -27.1512) -> (-3.1359, -27.3232)
  line L1666 (-3.1359, -27.3232) -> (-3.2282, -27.503)
  line L1667 (-3.2282, -27.503) -> (-3.3301, -27.6917)
  line L1668 (-3.3301, -27.6917) -> (-3.4414, -27.8879)
  line L1669 (-3.4414, -27.8879) -> (-3.563, -28.0921)
  line L1670 (-3.563, -28.0921) -> (-3.6691, -28.2628)
  arc A43 (-4.4421, -28.1517) -> (-3.6691, -28.2628) centre (0, 0) ccw
  line L1671 (-4.4421, -28.1517) -> (-4.4958, -27.958)
  line L1672 (-4.4958, -27.958) -> (-4.555, -27.7277)
  line L1673 (-4.555, -27.7277) -> (-4.6065, -27.5082)
  line L1674 (-4.6065, -27.5082) -> (-4.651, -27.2985)
  line L1675 (-4.651, -27.2985) -> (-4.6889, -27.0999)
  line L1676 (-4.6889, -27.0999) -> (-4.7208, -26.9113)
  line L1677 (-4.7208, -26.9113) -> (-4.7473, -26.7323)
  line L1678 (-4.7473, -26.7323) -> (-4.7684, -26.565)
  line L1679 (-4.7684, -26.565) -> (-4.7849, -26.4087)
  line L1680 (-4.7849, -26.4087) -> (-4.8056, -26.1272)
  line L1681 (-4.8056, -26.1272) -> (-4.8153, -25.816)
  line L1682 (-4.8153, -25.816) -> (-4.8231, -25.7385)
  line L1683 (-4.8231, -25.7385) -> (-4.8359, -25.6726)
  line L1684 (-4.8359, -25.6726) -> (-4.8534, -25.6186)
  line L1685 (-4.8534, -25.6186) -> (-4.875, -25.5768)
  line L1686 (-4.875, -25.5768) -> (-4.9003, -25.5471)
  line L1687 (-4.9003, -25.5471) -> (-4.9287, -25.5297)
  line L1688 (-4.9287, -25.5297) -> (-4.9629, -25.522)
  line L1689 (-4.9629, -25.522) -> (-5.1634, -25.4821)
  line L1690 (-5.1634, -25.4821) -> (-5.3636, -25.4408)
  line L1691 (-5.3636, -25.4408) -> (-5.398, -25.4346)
  line L1692 (-5.398, -25.4346) -> (-5.4309, -25.4395)
  line L1693 (-5.4309, -25.4395) -> (-5.4658, -25.4571)
  line L1694 (-5.4658, -25.4571) -> (-5.502, -25.4872)
  line L1695 (-5.502, -25.4872) -> (-5.5391, -25.5301)
  line L1696 (-5.5391, -25.5301) -> (-5.5766, -25.5858)
  line L1697 (-5.5766, -25.5858) -> (-5.6139, -25.6542)
  line L1698 (-5.6139, -25.6542) -> (-5.7439, -25.937)
  line L1699 (-5.7439, -25.937) -> (-5.8727, -26.1882)
  line L1700 (-5.8727, -26.1882) -> (-5.9487, -26.3259)
  line L1701 (-5.9487, -26.3259) -> (-6.0333, -26.4717)
  line L1702 (-6.0333, -26.4717) -> (-6.1273, -26.6263)
  line L1703 (-6.1273, -26.6263) -> (-6.2301, -26.7876)
  line L1704 (-6.2301, -26.7876) -> (-6.3423, -26.9558)
  line L1705 (-6.3423, -26.9558) -> (-6.465, -27.1316)
  line L1706 (-6.465, -27.1316) -> (-6.5979, -27.3138)
  line L1707 (-6.5979, -27.3138) -> (-6.742, -27.5029)
  line L1708 (-6.742, -27.5029) -> (-6.8669, -27.6604)
  arc A44 (-7.6222, -27.4618) -> (-6.8669, -27.6604) centre (0, 0) ccw
  line L1709 (-7.6222, -27.4618) -> (-7.6535, -27.2633)
  line L1710 (-7.6535, -27.2633) -> (-7.686, -27.0278)
  line L1711 (-7.686, -27.0278) -> (-7.7121, -26.8038)
  line L1712 (-7.7121, -26.8038) -> (-7.7325, -26.5903)
  line L1713 (-7.7325, -26.5903) -> (-7.7475, -26.3887)
  line L1714 (-7.7475, -26.3887) -> (-7.7577, -26.1977)
  line L1715 (-7.7577, -26.1977) -> (-7.7636, -26.0169)
  line L1716 (-7.7636, -26.0169) -> (-7.7655, -25.8483)
  line L1717 (-7.7655, -25.8483) -> (-7.764, -25.6911)
  line L1718 (-7.764, -25.6911) -> (-7.7526, -25.4091)
  line L1719 (-7.7526, -25.4091) -> (-7.7268, -25.0988)
  line L1720 (-7.7268, -25.0988) -> (-7.7256, -25.0209)
  line L1721 (-7.7256, -25.0209) -> (-7.7309, -24.954)
  line L1722 (-7.7309, -24.954) -> (-7.7421, -24.8984)
  line L1723 (-7.7421, -24.8984) -> (-7.7588, -24.8543)
  line L1724 (-7.7588, -24.8543) -> (-7.7805, -24.8219)
  line L1725 (-7.7805, -24.8219) -> (-7.8067, -24.8015)
  line L1726 (-7.8067, -24.8015) -> (-7.8398, -24.79)
  line L1727 (-7.8398, -24.79) -> (-8.0344, -24.7275)
  line L1728 (-8.0344, -24.7275) -> (-8.2286, -24.6636)
  line L1729 (-8.2286, -24.6636) -> (-8.2622, -24.6535)
  line L1730 (-8.2622, -24.6535) -> (-8.2954, -24.6546)
  line L1731 (-8.2954, -24.6546) -> (-8.332, -24.6681)
  line L1732 (-8.332, -24.6681) -> (-8.3714, -24.6939)
  line L1733 (-8.3714, -24.6939) -> (-8.4132, -24.7323)
  line L1734 (-8.4132, -24.7323) -> (-8.4568, -24.7833)
  line L1735 (-8.4568, -24.7833) -> (-8.5017, -24.8471)
  line L1736 (-8.5017, -24.8471) -> (-8.6631, -25.1132)
  line L1737 (-8.6631, -25.1132) -> (-8.8196, -25.3481)
  line L1738 (-8.8196, -25.3481) -> (-8.9108, -25.4762)
  line L1739 (-8.9108, -25.4762) -> (-9.0115, -25.6114)
  line L1740 (-9.0115, -25.6114) -> (-9.1225, -25.7543)
  line L1741 (-9.1225, -25.7543) -> (-9.243, -25.9028)
  line L1742 (-9.243, -25.9028) -> (-9.3737, -26.0571)
  line L1743 (-9.3737, -26.0571) -> (-9.5156, -26.2178)
  line L1744 (-9.5156, -26.2178) -> (-9.6684, -26.3836)
  line L1745 (-9.6684, -26.3836) -> (-9.8331, -26.5551)
  line L1746 (-9.8331, -26.5551) -> (-9.9752, -26.6973)
  arc A45 (-10.7029, -26.414) -> (-9.9752, -26.6973) centre (0, 0) ccw
  line L1747 (-10.7029, -26.414) -> (-10.7114, -26.2131)
  line L1748 (-10.7114, -26.2131) -> (-10.7168, -25.9755)
  line L1749 (-10.7168, -25.9755) -> (-10.7173, -25.75)
  line L1750 (-10.7173, -25.75) -> (-10.7132, -25.5356)
  line L1751 (-10.7132, -25.5356) -> (-10.7051, -25.3336)
  line L1752 (-10.7051, -25.3336) -> (-10.6935, -25.1426)
  line L1753 (-10.6935, -25.1426) -> (-10.6787, -24.9623)
  line L1754 (-10.6787, -24.9623) -> (-10.6614, -24.7946)
  line L1755 (-10.6614, -24.7946) -> (-10.642, -24.6386)
  line L1756 (-10.642, -24.6386) -> (-10.5985, -24.3597)
  line L1757 (-10.5985, -24.3597) -> (-10.5374, -24.0545)
  line L1758 (-10.5374, -24.0545) -> (-10.5274, -23.9771)
  line L1759 (-10.5274, -23.9771) -> (-10.525, -23.9101)
  line L1760 (-10.525, -23.9101) -> (-10.5298, -23.8536)
  line L1761 (-10.5298, -23.8536) -> (-10.5414, -23.8079)
  line L1762 (-10.5414, -23.8079) -> (-10.5593, -23.7732)
  line L1763 (-10.5593, -23.7732) -> (-10.583, -23.7499)
  line L1764 (-10.583, -23.7499) -> (-10.6145, -23.7347)
  line L1765 (-10.6145, -23.7347) -> (-10.8008, -23.6504)
  line L1766 (-10.8008, -23.6504) -> (-10.9864, -23.5649)
  line L1767 (-10.9864, -23.5649) -> (-11.0186, -23.551)
  line L1768 (-11.0186, -23.551) -> (-11.0518, -23.5483)
  line L1769 (-11.0518, -23.5483) -> (-11.0897, -23.5575)
  line L1770 (-11.0897, -23.5575) -> (-11.1318, -23.5787)
  line L1771 (-11.1318, -23.5787) -> (-11.1776, -23.6121)
  line L1772 (-11.1776, -23.6121) -> (-11.2267, -23.6578)
  line L1773 (-11.2267, -23.6578) -> (-11.2786, -23.716)
  line L1774 (-11.2786, -23.716) -> (-11.4693, -23.962)
  line L1775 (-11.4693, -23.962) -> (-11.6516, -24.1775)
  line L1776 (-11.6516, -24.1775) -> (-11.7568, -24.2943)
  line L1777 (-11.7568, -24.2943) -> (-11.8722, -24.4173)
  line L1778 (-11.8722, -24.4173) -> (-11.9988, -24.5465)
  line L1779 (-11.9988, -24.5465) -> (-12.1355, -24.6803)
  line L1780 (-12.1355, -24.6803) -> (-12.2829, -24.8187)
  line L1781 (-12.2829, -24.8187) -> (-12.4422, -24.9622)
  line L1782 (-12.4422, -24.9622) -> (-12.6129, -25.1096)
  line L1783 (-12.6129, -25.1096) -> (-12.7961, -25.2611)
  line L1784 (-12.7961, -25.2611) -> (-12.9534, -25.3862)
  arc A46 (-13.6441, -25.0218) -> (-12.9534, -25.3862) centre (0, 0) ccw
  line L1785 (-13.6441, -25.0218) -> (-13.6296, -24.8213)
  line L1786 (-13.6296, -24.8213) -> (-13.608, -24.5845)
  line L1787 (-13.608, -24.5845) -> (-13.5827, -24.3604)
  line L1788 (-13.5827, -24.3604) -> (-13.5542, -24.1479)
  line L1789 (-13.5542, -24.1479) -> (-13.5231, -23.9481)
  line L1790 (-13.5231, -23.9481) -> (-13.4898, -23.7598)
  line L1791 (-13.4898, -23.7598) -> (-13.4546, -23.5824)
  line L1792 (-13.4546, -23.5824) -> (-13.4182, -23.4177)